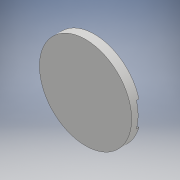
# Autodesk Inventor part: Diffuser_V1
Saved by Autodesk Inventor 2018 (Build 220112000, 112)
## iProperties
Created: 2017-07-21
Part Number: Diffuser_V1
Material: Generic
Document SubType Name: Modeling
Designer: Micha
Density: 1 g/cm^3
Appearance: Default
Author: Micha
Autodesk Inventor part; units mm, degrees
ref_plane "YZ Plane" through (0, 0, 0) normal (1, 0, 0) x (0, 1, 0)
ref_plane "XZ Plane" through (0, 0, 0) normal (0, 1, 0) x (-1, 0, 0)
ref_plane "XY Plane" through (0, 0, 0) normal (0, 0, 1) x (1, 0, 0)
sketch "Sketch1" plane through (0, 0, 0) normal (0, 1, 0) x (-1, 0, 0)
  circle A0 centre (0, 0) radius 28
  dimension "d7" = 56
  constraints: 1 centre point
  measures "d7" diameter of A0
extrude "Extrusion1" add sketch "Sketch1" along normal blind 0.4
sketch "Sketch2" plane through (0, 0.4, 0) normal (0, 1, 0) x (1, 0, 0)
  circle A0 centre (0, 0) radius 27.25
  circle A1 centre (0, 0) radius 28
  dimension "d4" = 54.5
  dimension "d8" = 56
  constraints: 2 centre point, 1 coincident
  measures "d4" diameter of A0
  measures "d8" diameter of A1
extrude "Extrusion2" add sketch "Sketch2" along normal blind 5
sketch "Sketch3" plane through (0, 5.4, 0) normal (0, 1, 0) x (1, 0, 0)
  arc A0 (-15.63, 22.3219) -> (-17.149, 21.1772) centre (0, 0) ccw
  line L0 (0, 0) -> (-17.149, 21.1772) construction
  line L1 (0, 0) -> (27.25, 0) construction
  line L2 (0, 0) -> (-15.63, 22.3219) construction
  arc A1 (-15.0564, 21.5027) -> (-16.5197, 20.4001) centre (0, 0) ccw
  line L3 (0, 0) -> (-16.5197, 20.4001) construction
  line L4 (0, 0) -> (26.25, 0) construction
  line L5 (0, 0) -> (-15.0564, 21.5027) construction
  line L6 (-16.5197, 20.4001) -> (-17.149, 21.1772)
  line L7 (-15.0564, 21.5027) -> (-15.63, 22.3219)
  circle A2 centre (0, 0) radius 27.25 projected
  dimension "d9" = 27.25
  dimension "d10" = 129
  dimension "d11" = 4
  dimension "d12" = 26.25
  dimension "d13" = 129
  dimension "d14" = 4
  constraints: 16 end point, 5 point on circle, 2 centre point, 2 coincident, 2 equal length, 2 horizontal, 1 point on line
  measures "d9" radius of A0
  measures "d10" angle of L1 L0
  measures "d11" angle of L2 L0
  measures "d12" radius of A1
  measures "d13" angle of L4 L3
  measures "d14" angle of L5 L3
extrude "Extrusion3" add sketch "Sketch3" against normal blind 1.4 contours L7 A1 L6 A0
fillet "Fillet1" radius 0.5 4 edges at (-15.3432, 4, -21.9123) (-15.3432, 5.4, -21.9123) (-16.8343, 5.4, -20.7887) (-16.8343, 4, -20.7887)
pattern_circular "Circular Pattern1" count 2 over 360 about axis through (0, 0, 0) along (0, 1, 0) of "Extrusion3", "Fillet1"
sketch "Sketch4" plane through (0, 5.4, 0) normal (0, 1, 0) x (1, 0, 0)
  circle A0 centre (0, 0) radius 28 projected
  line L0 (0, 28) -> (-7.5, 28)
  line L1 (-7.5, 28) -> (-7.5, 25)
  line L2 (-7.5, 25) -> (0, 25)
  line L3 (0, 25) -> (0, 28)
  line L4 (0, 25) -> (7.5, 25)
  line L5 (7.5, 25) -> (7.5, 28)
  line L6 (7.5, 28) -> (0, 28)
  line L7 (0, 28) -> (0, 25)
  circle A1 centre (0, 0) radius 28 projected
  line L8 (28, 0) -> (25, 0)
  line L9 (25, 0) -> (25, 7.5)
  line L10 (25, 7.5) -> (28, 7.5)
  line L11 (28, 7.5) -> (28, 0)
  line L12 (28, 0) -> (25, 0)
  line L13 (25, 0) -> (25, -7.5)
  line L14 (25, -7.5) -> (28, -7.5)
  line L15 (28, -7.5) -> (28, 0)
  dimension "d25" = 7.5
  dimension "d26" = 3
  dimension "d27" = 7.5
  dimension "d28" = 3
  dimension "d51" = 3
  dimension "d52" = 7.5
  dimension "d53" = 3
  dimension "d54" = 7.5
  constraints: 32 end point, 8 parallel, 4 perpendicular
  measures "d25" distance of L2.end L1.end
  measures "d26" distance of L1.end L0.end
  measures "d27" distance of L6.end L5.end
  measures "d28" distance of L5.end L4.end
  measures "d51" distance of L9.end L10.end
  measures "d52" distance of L8.end L9.end
  measures "d53" distance of L14.end L13.end
  measures "d54" distance of L13.end L12.end
extrude "Extrusion4" cut sketch "Sketch4" against normal blind 1.5 contours L8 L9 L10 A0 | L15 L14 A0 | A0 L14 L13 L8 | A0 L10 L11 | L5 L4 L3 A0 | A0 L6 L5 | L1 L0 A0 | A0 L3 L2 L1
sketch "Sketch7" plane through (0, 0.4, 0) normal (0, 1, 0) x (1, 0, 0)
  circle A0 centre (0, 0) radius 24
  circle A1 centre (0, 0) radius 27.25
  dimension "d47" = 48
  dimension "d50" = 54.5
  constraints: 2 centre point, 2 coincident
  measures "d47" diameter of A0
  measures "d50" diameter of A1
extrude "Extrusion7" add sketch "Sketch7" along normal blind 1.5
body "Solid1"
